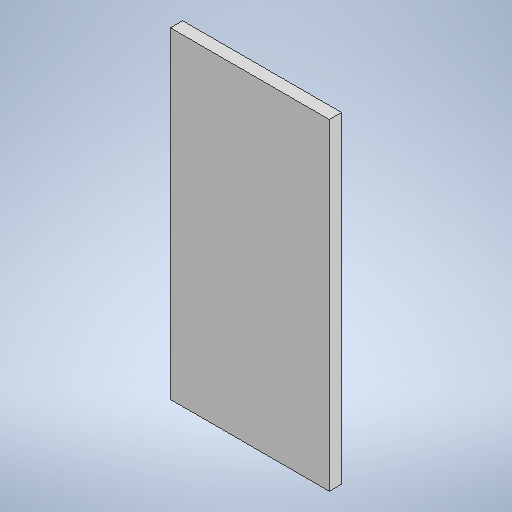
# Autodesk Inventor part: Door
Saved by Autodesk Inventor 2026.2 (Build 302298010, 298A)
## iProperties
Created: 2026-03-19
Part Number: Door
Material: Ogólny
Document SubType Name: Modeling
Designer: Patryk
Density: 1 g/cm^3
Appearance: Domyślna
Author: Patryk
Autodesk Inventor part; units mm, degrees
ref_plane "YZ Plane" through (0, 0, 0) normal (1, 0, 0) x (0, 1, 0)
ref_plane "XZ Plane" through (0, 0, 0) normal (0, 1, 0) x (-1, 0, 0)
ref_plane "XY Plane" through (0, 0, 0) normal (0, 0, 1) x (1, 0, 0)
sketch "Szkic1" plane through (0, 0, 0) normal (0, 0, 1) x (1, 0, 0)
  line L0 (39, 79) -> (-39, 79)
  line L1 (-39, 79) -> (-39, -79)
  line L2 (-39, -79) -> (39, -79)
  line L3 (39, -79) -> (39, 79)
  line L4 (39, 79) -> (-39, -79) construction
  line L5 (-39, 79) -> (39, -79) construction
  point P0 (0, 0)
  dimension "d0" = 78
  dimension "d1" = 158
  constraints: 12 end point, 2 midpoint, 2 parallel, 1 horizontal, 1 perpendicular
  measures "d0" distance of L2.end L1.end
  measures "d1" distance of L1.end L0.end
extrude "Wyciągnięcie proste1" add sketch "Szkic1" along normal mid plane 6
